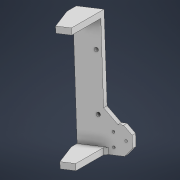
# Autodesk Inventor part: psu holder right
Saved by Autodesk Inventor 2021 (Build 250183000, 183)
## iProperties
Created: 2020-10-29
Part Number: psu holder right
Material: Generic
Document SubType Name: Modeling
Designer: brand
Density: 1 g/cm^3
Appearance: Default
Author: brand
## iProperties of the stored document _3DPrint.ipt
Created: 2020-10-29
Part Number: _3DPrint
Material: Generic
Document SubType Name: Modeling
Designer: brand
Density: 1 g/cm^3
Appearance: Default
Author: brand
Autodesk Inventor part; units mm, degrees
ref_plane "YZ Plane" through (0, 0, 0) normal (1, 0, 0) x (0, 1, 0)
ref_plane "XZ Plane" through (0, 0, 0) normal (0, 1, 0) x (-1, 0, 0)
ref_plane "XY Plane" through (0, 0, 0) normal (0, 0, 1) x (1, 0, 0)
derived "psu holder left.ipt"
sketch "Sketch1" plane through (0, 0, 0) normal (0, 0, 1) x (1, 0, 0)
  line L0 (0, 25) -> (-25, 25)
  line L1 (-25, 25) -> (-25, -25)
  line L2 (-25, -25) -> (0, -25)
  line L3 (0, -25) -> (0, 25)
  line L4 (-30, 0) -> (5, 0) projected
  line L5 (0, -35) -> (0, 35) projected
  point P0 (0, 0)
  dimension "d1" = 25
  dimension "d2" = 25
  dimension "d3" = 25
  constraints: 8 end point, 2 parallel, 1 collinear, 1 horizontal, 1 perpendicular
  measures "d1" distance between parallel lines of L4 L0
  measures "d2" distance between parallel lines of L2 L4
  measures "d3" distance of L0.start L0.end
extrude "Extrusion1" add sketch "Sketch1" along normal blind 6
sketch "Sketch2" plane through (0, 0, 0) normal (0, 0, 1) x (1, 0, 0)
  line L0 (0, 25) -> (-25, 25) projected
  line L1 (0, 25) -> (-25, 25) projected
  line L2 (-25, 25) -> (-25, 31)
  line L3 (-25, 31) -> (0, 31)
  line L4 (0, 31) -> (0, 25)
  point P0 (0, 0)
  point P1 (0, -25)
  point P2 (-25, -25)
  dimension "d10" = 6
  constraints: 6 end point, 2 perpendicular, 1 vertical
  measures "d10" distance of L3.end L0.start
extrude "Extrusion2" add sketch "Sketch2" along normal blind 59.5
mirror "Mirror1" about plane through (-12.5, 28, 59.5) normal (0, 0, 1) of "Extrusion1", "Extrusion2"
sketch "Sketch3" plane through (-25, 31, 0) normal (0, 1, 0) x (1, 0, 0)
  line L0 (25, 0) -> (0, 0) construction
  line L1 (25, 0) -> (25, -119) construction
  line L2 (25, 0) -> (50, 0)
  line L3 (50, -26) -> (25, -26)
  line L4 (25, -26) -> (25, 0)
  line L5 (50, -26) -> (50, 0)
  line L6 (58.0605, -13) -> (16.897, -13) construction
  line L7 (37, -29.747) -> (37, 7.436) construction
  circle A0 centre (37, -13) radius 7.5 construction
  circle A1 centre (44.5, -13) radius 1.25
  circle A2 centre (33.25, -6.5048) radius 1.25
  circle A3 centre (33.25, -19.4952) radius 1.25
  dimension "d17" = 15
  dimension "d13" = 25
  dimension "d14" = 26
  dimension "d15" = 13
  dimension "d16" = 12
  dimension "d18" = 2.5
  dimension "d21" = 360
  constraints: 12 end point, 4 point on line, 3 centre point, 2 horizontal, 2 vertical, 1 horizontal alignment, 1 parallel, 1 perpendicular, 9 other
  measures "d13" distance of L3.start L3.end
  measures "d14" distance of L3.start L2.end
  measures "d15" distance between parallel lines of L3 L6
  measures "d16" distance between parallel lines of L7 L1
  measures "d18" diameter of A1
extrude "Extrusion3" add sketch "Sketch3" against normal blind 6
chamfer "Chamfer1" distance 7.5 angle 45 2 edges at (25, 28, 26) (25, 28, 0)
chamfer "Chamfer2" distance 12.5 angle 45 1 edges at (0, 28, 26)
chamfer "Chamfer3" distance 3 angle 45 1 edges at (0, 25, 3)
chamfer "Chamfer4" distance 40 angle 15 2 edges at (-25, -25, 116) (-25, -25, 3) measured on face at (-25, -24.5, 3) measured on face at (-25, -24.5, 116)
sketch "Sketch4" plane through (-25, 25, 113) normal (0, -1, 0) x (1, 0, 0)
  line L0 (25, -74.5) -> (25, 0) projected
  line L1 (20, 10.7001) -> (20, -118.0828) construction
  circle A0 centre (20, -26.5) radius 2
  circle A1 centre (20, -80.5) radius 2
  line L2 (10.718, 0) -> (25, 0) construction
  line L3 (10.718, -107) -> (25, -107) construction
  point P0 (25, -113)
  dimension "d37" = 5
  dimension "d38" = 4
  dimension "d39" = 4
  dimension "d40" = 54
  dimension "d41" = 26.5
  dimension "d42" = 26.5
  constraints: 2 centre point, 2 end point, 2 point on line, 1 vertical
  measures "d37" distance between parallel lines of L0 L1
  measures "d38" diameter of A0
  measures "d39" diameter of A1
  measures "d40" distance of A1.centre A0.centre
  measures "d41" distance from line of L2 A0.centre
  measures "d42" distance from line of L3 A1.centre
extrude "Extrusion4" cut sketch "Sketch4" against normal through all
equation "\"d1\" = 0.5 * depth"
equation "\"d2\" = d1"
equation "\"d4\" = wall_thickness"
equation "\"d10\" = wall_thickness"
equation "\"d11\" = wall_thickness + 0.5 * width"
equation "\"d15\" = 0.5 * d14"
equation "\"d23\" = wall_thickness"
equation "\"d41\" = d42"
equation "\"depth\" = 50"
equation "\"wall_thickness\" = 6"
equation "\"width\" = 107"
body "Solid1"
